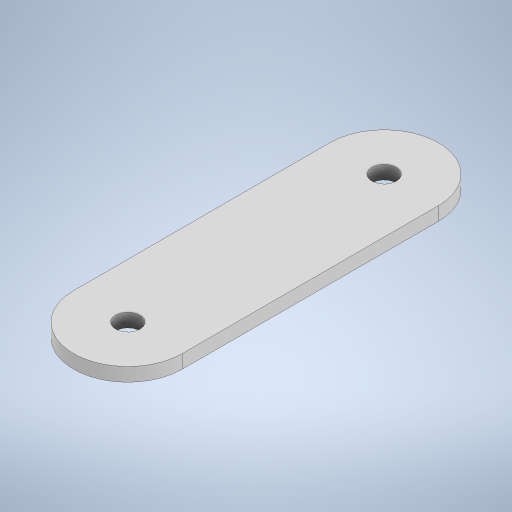
# Autodesk Inventor part: ベルト
Saved by Autodesk Inventor 2024.1 (Build 281209000, 209)
## iProperties
Created: 2024-03-26
Part Number: ベルト
Material: 一般
Document SubType Name: Modeling
Designer: hibik
Density: 1 g/cm^3
Appearance: 既定
Author: hibik
Autodesk Inventor part; units mm, degrees
ref_plane "YZ Plane" through (0, 0, 0) normal (1, 0, 0) x (0, 1, 0)
ref_plane "XZ Plane" through (0, 0, 0) normal (0, 1, 0) x (-1, 0, 0)
ref_plane "XY Plane" through (0, 0, 0) normal (0, 0, 1) x (1, 0, 0)
sketch "スケッチ1" plane through (0, 0, 0) normal (0, 1, 0) x (-1, 0, 0)
  line L0 (0, 0) -> (20, 0) construction
  line L1 (20, 0) -> (20, -47.1)
  line L2 (20, -47.1) -> (0, -47.1) construction
  line L3 (0, -47.1) -> (0, 0)
  circle A0 centre (10, 0) radius 10
  circle A1 centre (10, -47.1) radius 10
  circle A2 centre (10, 0) radius 2.25
  circle A3 centre (10, -47.1) radius 2.25
  dimension "d0" = 47.1
  dimension "d1" = 20
  dimension "d4" = 4.5
  dimension "d5" = 4.5
  constraints: 8 end point, 2 centre point, 2 coincident, 2 midpoint, 2 parallel, 1 horizontal, 1 perpendicular, 6 other
  measures "d0" distance of L0.end L1.end
  measures "d1" distance of L0.start L0.end
  measures "d4" diameter of A2
  measures "d5" diameter of A3
extrude "押し出し1" add sketch "スケッチ1" along normal blind 2.5
